Autodesk Fusion 360 part; units mm, degrees
(part 3 of 3)
  spline S126 degree 2 poles (33.1299, -35.2235) (34.2042, -35.7863) (34.7312, -36.6202) knots 0 0 0 1 1 1
  spline S127 degree 2 poles (34.7312, -36.6202) (35.2581, -37.4541) (35.2581, -38.4875) knots 0 0 0 1 1 1
  spline S128 degree 2 poles (35.2581, -38.4875) (35.2581, -39.6232) (34.6135, -40.6106) knots 0 0 0 1 1 1
  spline S129 degree 2 poles (34.6135, -40.6106) (33.9689, -41.598) (32.7308, -42.1096) knots 0 0 0 1 1 1
  spline S130 degree 2 poles (32.7308, -42.1096) (31.4928, -42.6212) (29.9785, -42.6212) knots 0 0 0 1 1 1
  spline S131 degree 2 poles (29.9785, -42.6212) (28.3106, -42.6212) (27.0368, -42.084) knots 0 0 0 1 1 1
  spline S132 degree 2 poles (27.0368, -42.084) (25.7629, -41.5468) (25.0774, -40.5032) knots 0 0 0 1 1 1
  spline S133 degree 2 poles (25.0774, -40.5032) (24.3918, -39.4595) (24.3407, -38.1396) knots 0 0 0 1 1 1
  line L79 (24.3407, -38.1396) -> (26.2438, -37.9964)
  spline S134 degree 2 poles (26.2438, -37.9964) (26.3973, -39.4186) (27.2823, -40.1451) knots 0 0 0 1 1 1
  spline S135 degree 2 poles (27.2823, -40.1451) (28.1674, -40.8715) (29.8966, -40.8715) knots 0 0 0 1 1 1
  spline S136 degree 2 poles (29.8966, -40.8715) (31.6974, -40.8715) (32.5211, -40.2116) knots 0 0 0 1 1 1
  spline S137 degree 2 poles (32.5211, -40.2116) (33.3448, -39.5516) (33.3448, -38.6205) knots 0 0 0 1 1 1
  spline S138 degree 2 poles (33.3448, -38.6205) (33.3448, -37.8122) (32.7615, -37.2904) knots 0 0 0 1 1 1
  spline S139 degree 2 poles (32.7615, -37.2904) (32.1885, -36.7685) (29.7687, -36.2211) knots 0 0 0 1 1 1
  spline S140 degree 2 poles (29.7687, -36.2211) (27.3488, -35.6737) (26.4484, -35.2644) knots 0 0 0 1 1 1
  spline S141 degree 2 poles (26.4484, -35.2644) (25.1387, -34.6608) (24.5146, -33.7348) knots 0 0 0 1 1 1
  spline S142 degree 2 poles (24.5146, -33.7348) (23.8905, -32.8088) (23.8905, -31.6014) knots 0 0 0 1 1 1
  spline S143 degree 2 poles (23.8905, -31.6014) (23.8905, -30.4043) (24.576, -29.3453) knots 0 0 0 1 1 1
  spline S144 degree 2 poles (24.576, -29.3453) (25.2615, -28.2863) (26.5456, -27.6979) knots 0 0 0 1 1 1
  spline S145 degree 2 poles (26.5456, -27.6979) (27.8297, -27.1096) (29.4362, -27.1096) knots 0 0 0 1 1 1
  spline S146 degree 2 poles (29.4362, -27.1096) (31.4723, -27.1096) (32.8485, -27.703) knots 0 0 0 1 1 1
  spline S147 degree 2 poles (32.8485, -27.703) (34.2247, -28.2965) (35.0074, -29.4885) knots 0 0 0 1 1 1
  spline S148 degree 2 poles (35.0074, -29.4885) (35.7902, -30.6805) (35.8311, -32.1846) knots 0 0 0 1 1 1
  line L80 (21.2404, -27.3654) -> (21.2404, -42.3654)
  line L81 (21.2404, -42.3654) -> (18.2527, -42.3654)
  line L82 (18.2527, -42.3654) -> (14.7022, -31.7447)
  spline S149 degree 2 poles (14.7022, -31.7447) (14.2111, -30.261) (13.986, -29.5243) knots 0 0 0 1 1 1
  spline S150 degree 2 poles (13.986, -29.5243) (13.7302, -30.3429) (13.1879, -31.9288) knots 0 0 0 1 1 1
  line L83 (13.1879, -31.9288) -> (9.5965, -42.3654)
  line L84 (9.5965, -42.3654) -> (6.9259, -42.3654)
  line L85 (6.9259, -42.3654) -> (6.9259, -27.3654)
  line L86 (6.9259, -27.3654) -> (8.8393, -27.3654)
  line L87 (8.8393, -27.3654) -> (8.8393, -39.92)
  line L88 (8.8393, -39.92) -> (13.1981, -27.3654)
  line L89 (13.1981, -27.3654) -> (14.9887, -27.3654)
  line L90 (14.9887, -27.3654) -> (19.327, -40.1348)
  line L91 (19.327, -40.1348) -> (19.327, -27.3654)
  line L92 (19.327, -27.3654) -> (21.2404, -27.3654)
  line L93 (5.3707, -27.3654) -> (-0.3899, -42.3654)
  line L94 (-0.3899, -42.3654) -> (-2.5284, -42.3654)
  line L95 (-2.5284, -42.3654) -> (-8.6675, -27.3654)
  line L96 (-8.6675, -27.3654) -> (-6.4063, -27.3654)
  line L97 (-6.4063, -27.3654) -> (-4.6566, -31.9084)
  line L98 (-4.6566, -31.9084) -> (1.6156, -31.9084)
  line L99 (1.6156, -31.9084) -> (3.2629, -27.3654)
  line L100 (3.2629, -27.3654) -> (5.3707, -27.3654)
  line L101 (1.0426, -33.525) -> (-4.0427, -33.525)
  line L102 (-4.0427, -33.525) -> (-2.4772, -37.6792)
  spline S151 degree 2 poles (-2.4772, -37.6792) (-1.761, -39.5721) (-1.4131, -40.7897) knots 0 0 0 1 1 1
  spline S152 degree 2 poles (-1.4131, -40.7897) (-1.1266, -39.347) (-0.6048, -37.9247) knots 0 0 0 1 1 1
  line L103 (-0.6048, -37.9247) -> (1.0426, -33.525)
  line L104 (-10.2842, -27.3654) -> (-10.2842, -42.3654)
  line L105 (-10.2842, -42.3654) -> (-16.9349, -42.3654)
  spline S153 degree 2 poles (-16.9349, -42.3654) (-18.9404, -42.3654) (-19.984, -41.9612) knots 0 0 0 1 1 1
  spline S154 degree 2 poles (-19.984, -41.9612) (-21.0277, -41.5571) (-21.6518, -40.5339) knots 0 0 0 1 1 1
  spline S155 degree 2 poles (-21.6518, -40.5339) (-22.276, -39.5107) (-22.276, -38.2726) knots 0 0 0 1 1 1
  spline S156 degree 2 poles (-22.276, -38.2726) (-22.276, -36.6764) (-21.2426, -35.5816) knots 0 0 0 1 1 1
  spline S157 degree 2 poles (-21.2426, -35.5816) (-20.2091, -34.4868) (-18.0502, -34.1901) knots 0 0 0 1 1 1
  spline S158 degree 2 poles (-18.0502, -34.1901) (-18.8381, -33.8115) (-19.2473, -33.4432) knots 0 0 0 1 1 1
  spline S159 degree 2 poles (-19.2473, -33.4432) (-20.117, -32.6451) (-20.8947, -31.4479) knots 0 0 0 1 1 1
  line L106 (-20.8947, -31.4479) -> (-23.5038, -27.3654)
  line L107 (-23.5038, -27.3654) -> (-21.0072, -27.3654)
  line L108 (-21.0072, -27.3654) -> (-19.0222, -30.4861)
  spline S160 degree 2 poles (-19.0222, -30.4861) (-18.1525, -31.8367) (-17.5898, -32.553) knots 0 0 0 1 1 1
  spline S161 degree 2 poles (-17.5898, -32.553) (-17.027, -33.2692) (-16.5819, -33.5557) knots 0 0 0 1 1 1
  spline S162 degree 2 poles (-16.5819, -33.5557) (-16.1368, -33.8422) (-15.6764, -33.9547) knots 0 0 0 1 1 1
  spline S163 degree 2 poles (-15.6764, -33.9547) (-15.3387, -34.0264) (-14.5713, -34.0264) knots 0 0 0 1 1 1
  line L109 (-14.5713, -34.0264) -> (-12.2692, -34.0264)
  line L110 (-12.2692, -34.0264) -> (-12.2692, -27.3654)
  line L111 (-12.2692, -27.3654) -> (-10.2842, -27.3654)
  line L112 (-12.2692, -35.7453) -> (-16.5359, -35.7453)
  spline S164 degree 2 poles (-16.5359, -35.7453) (-17.8967, -35.7453) (-18.6641, -36.0267) knots 0 0 0 1 1 1
  spline S165 degree 2 poles (-18.6641, -36.0267) (-19.4315, -36.3081) (-19.8306, -36.9271) knots 0 0 0 1 1 1
  spline S166 degree 2 poles (-19.8306, -36.9271) (-20.2296, -37.5462) (-20.2296, -38.2726) knots 0 0 0 1 1 1
  spline S167 degree 2 poles (-20.2296, -38.2726) (-20.2296, -39.3367) (-19.4571, -40.0223) knots 0 0 0 1 1 1
  spline S168 degree 2 poles (-19.4571, -40.0223) (-18.6846, -40.7078) (-17.0168, -40.7078) knots 0 0 0 1 1 1
  line L113 (-17.0168, -40.7078) -> (-12.2692, -40.7078)
  line L114 (-12.2692, -40.7078) -> (-12.2692, -35.7453)
  line L115 (-28.8244, -27.3654) -> (-28.8244, -40.5953)
  line L116 (-28.8244, -40.5953) -> (-23.8824, -40.5953)
  line L117 (-23.8824, -40.5953) -> (-23.8824, -42.3654)
  line L118 (-23.8824, -42.3654) -> (-35.7719, -42.3654)
  line L119 (-35.7719, -42.3654) -> (-35.7719, -40.5953)
  line L120 (-35.7719, -40.5953) -> (-30.8094, -40.5953)
  line L121 (-30.8094, -40.5953) -> (-30.8094, -27.3654)
  line L122 (-30.8094, -27.3654) -> (-28.8244, -27.3654)
extrude "Extrude26" cut sketch "Sketch23" against normal blind 3 contours L4 L5 L6 L7 L8 L9 L10 L11 | L12 L13 L14 L15 L16 L17 L18 L19 L20 L21 L22 L23 | L24 S0 S1 S2 S3 S4 S5 S6 S7 S8 S9 L25 S10 S11 S12 S13 S14 S15 S16 S17 S18 S19 | L26 L27 L28 L29 L30 L31 L32 L33 L34 L35 L36 L37 | L38 L39 L40 L41 L42 L43 L44 L45 L46 L47 | S20 S21 S22 S23 S24 S25 S26 S27 S28 S29 S30 | L48 L49 L50 L51 L52 L53 | S40 S41 S42 S43 S44 S45 S46 S47 S48 S49 S50 | L54 L55 L56 S60 S61 S62 S63 S64 S65 S66 S67 S68 S69 S70 L57 S71 S72 S73 S74 S75 S76 S77 S78 S79 S80 S81 S82 L58 L59 | L60 L61 L62 L63 | L64 L65 L66 L67 L68 L69 L70 L71 L72 L73 L74 L75 | L76 S83 S84 S85 S86 S87 S88 S89 S90 S91 S92 S93 S94 S95 S96 S97 S98 S99 S100 L77 S101 S102 S103 S104 S105 S106 S107 S108 S109 S110 S111 S112 S113 S114 S115 | L78 S116 S117 S118 S119 S120 S121 S122 S123 S124 S125 S126 S127 S128 S129 S130 S131 S132 S133 L79 S134 S135 S136 S137 S138 S139 S140 S141 S142 S143 S144 S145 S146 S147 S148 | L80 L81 L82 S149 S150 L83 L84 L85 L86 L87 L88 L89 L90 L91 L92 | L93 L94 L95 L96 L97 L98 L99 L100 | L104 L105 S153 S154 S155 S156 S157 S158 S159 L106 L107 L108 S160 S161 S162 S163 L109 L110 L111 | L115 L116 L117 L118 L119 L120 L121 L122 bodies 7 2 4 5 6 8 in component "BOX"
component "Stepper Motor" placed x (0, 0, -1) y (0, 1, 0) z (1, 0, 0) at (35.9133, 13.8869, 23.5505)
component "BOX" placed x (1, 0, 0) y (0, 1, 0) z (0, 0, 1) at (-4.0867, -19.4631, -4.2995)
component "LID" placed x (1, 0, 0) y (0, 1, 0) z (0, 0, 1) at (0, 0, -20)
